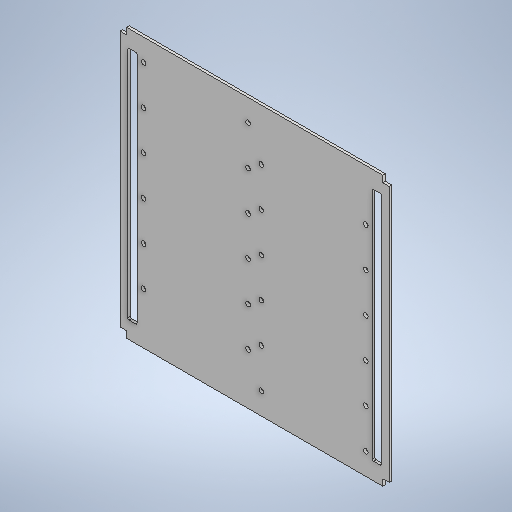
# Autodesk Inventor part: Baseplate_for_PCBs_mirroredHoles
Saved by Autodesk Inventor 2025.1 (Build 291241000, 241)
## iProperties
Created: 2025-04-15
Part Number: Baseplate_for_PCBs_mirroredHoles
Material: Generic
Document SubType Name: Modeling
Designer: edward.horrocks
Density: 1 g/cm^3
Appearance: Default
Author: edward.horrocks
Autodesk Inventor part; units mm, degrees
ref_plane "YZ Plane" through (0, 0, 0) normal (1, 0, 0) x (0, 1, 0)
ref_plane "XZ Plane" through (0, 0, 0) normal (0, 1, 0) x (-1, 0, 0)
ref_plane "XY Plane" through (0, 0, 0) normal (0, 0, 1) x (1, 0, 0)
sketch "Sketch2" plane through (0, 0, 0) normal (0, 0, 1) x (1, 0, 0)
  line L0 (-103, 103) -> (103, 103)
  line L1 (103, 103) -> (103, -103)
  line L2 (103, -103) -> (-103, -103)
  line L3 (-103, -103) -> (-103, 103)
  line L4 (-103, 103) -> (103, -103) construction
  line L5 (103, 103) -> (-103, -103) construction
  line L6 (-103, 103) -> (-98, 103)
  line L7 (-98, 103) -> (-98, 98)
  line L8 (-98, 98) -> (-103, 98)
  line L9 (-103, 98) -> (-103, 103)
  line L10 (103, 103) -> (98, 103)
  line L11 (98, 103) -> (98, 98)
  line L12 (98, 98) -> (103, 98)
  line L13 (103, 98) -> (103, 103)
  line L14 (103, -103) -> (98, -103)
  line L15 (98, -103) -> (98, -98)
  line L16 (98, -98) -> (103, -98)
  line L17 (103, -98) -> (103, -103)
  line L18 (-103, -103) -> (-98, -103)
  line L19 (-98, -103) -> (-98, -98)
  line L20 (-98, -98) -> (-103, -98)
  line L21 (-103, -98) -> (-103, -103)
  line L22 (90, 89) -> (90, -89)
  line L23 (-90, 90) -> (90, -90) construction
  line L24 (90, 90) -> (-90, -90) construction
  line L25 (-91, 90) -> (-96, 90)
  line L26 (-97, 89) -> (-97, -89)
  line L27 (-96, -90) -> (-91, -90)
  line L28 (-90, -89) -> (-90, 89)
  line L29 (91, 90) -> (96, 90)
  line L30 (97, 89) -> (97, -89)
  line L31 (96, -90) -> (91, -90)
  arc A0 (-96, 90) -> (-97, 89) centre (-96, 89) ccw
  arc A1 (-90, 89) -> (-91, 90) centre (-91, 89) ccw
  arc A2 (-91, -90) -> (-90, -89) centre (-91, -89) ccw
  arc A3 (-97, -89) -> (-96, -90) centre (-96, -89) ccw
  arc A4 (97, 89) -> (96, 90) centre (96, 89) ccw
  arc A5 (91, 90) -> (90, 89) centre (91, 89) ccw
  arc A6 (96, -90) -> (97, -89) centre (96, -89) ccw
  arc A7 (90, -89) -> (91, -90) centre (91, -89) ccw
  point P0 (0, 0)
  point P1 (-97, -90)
  point P2 (97, -90)
  dimension "d0" = 206
  dimension "d1" = 206
  dimension "d2" = 5
  dimension "d3" = 5
  dimension "d4" = 5
  dimension "d5" = 5
  dimension "d6" = 5
  dimension "d7" = 5
  dimension "d8" = 5
  dimension "d9" = 5
  dimension "d10" = 180
  dimension "d11" = 180
  dimension "d12" = 7
  dimension "d14" = 1
  dimension "d15" = 180
  constraints: 64 end point, 16 point on circle, 16 tangent, 13 parallel, 12 point on line, 8 centre point, 7 equal radius, 7 horizontal, 7 perpendicular, 4 midpoint
  measures "d0" distance of L1.end L2.end
  measures "d1" distance of L0.end L1.end
  measures "d2" distance of L7.end L8.end
  measures "d3" distance of L6.end L7.end
  measures "d4" distance of L12.end L11.end
  measures "d5" distance of L11.end L10.end
  measures "d6" distance of L15.end L16.end
  measures "d7" distance of L14.end L15.end
  measures "d8" distance of L20.end L19.end
  measures "d9" distance of L19.end L18.end
  measures "d10" distance of L23.end L24.end
  measures "d11" distance of L24.start L23.end
  measures "d12" distance of point (-90, -90) point (-97, -90)
  measures "d14" radius of A0
  measures "d15" distance between parallel lines of L22 L28
extrude "Extrusion1" add sketch "Sketch2" along normal blind 2 contours L0 L11 L12 L1 L16 L15 L2 L19 L20 L3 L8 L7
sketch "Sketch3" plane through (0, 0, 2) normal (0, 0, 1) x (1, 0, 0)
  circle A0 centre (-85, 86.25) radius 1.825
  point P0 (0, 0)
  dimension "d18" = 3.65
  constraints: 1 centre point
  measures "d18" diameter of A0
hole "Hole1" at (-85, 86.25, 2) direction (0, 0, -1) diameter 3.6 depth 10
pattern_linear "Rectangular Pattern1" count 2 spacing 80 along (1, 0, 0) count 6 spacing 30 along (0, -1, 0) of "Hole1"
sketch "Sketch4" plane through (0, 0, 2) normal (0, 0, 1) x (1, 0, 0)
  circle A0 centre (5, 63.75) radius 1.8
  line L0 (98, 103) -> (-98, 103) projected
  point P0 (0, 0)
  dimension "d33" = 3.6
  dimension "d47" = 39.25
  constraints: 1 centre point
  measures "d33" diameter of A0
  measures "d47" distance from line of L0 A0.centre
hole "Hole2" at (5, 63.75, 2) direction (0, 0, -1) diameter 3.6 depth 10
pattern_linear "Rectangular Pattern2" count 2 spacing 80 along (1, 0, 0) count 6 spacing 30 along (0, -1, 0) of "Hole2"
body "Solid1"
